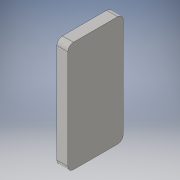
# Autodesk Inventor part: Phone
Saved by Autodesk Inventor 2016 (Build 200138000, 138)
## iProperties
Created: 2017-01-27
Part Number: Phone
Material: Generic
Document SubType Name: Modeling
Designer: RoboticsUser
Density: 1 g/cm^3
Appearance: Default
Author: RoboticsUser
Autodesk Inventor part; units mm, degrees
ref_plane "YZ Plane" through (0, 0, 0) normal (1, 0, 0) x (0, 1, 0)
ref_plane "XZ Plane" through (0, 0, 0) normal (0, 1, 0) x (-1, 0, 0)
ref_plane "XY Plane" through (0, 0, 0) normal (0, 0, 1) x (1, 0, 0)
sketch "Sketch1" plane through (0, 0, 0) normal (1, 0, 0) x (0, 1, 0)
  line L0 (0, 0) -> (127, 0)
  line L1 (127, 0) -> (127, -63.5)
  line L2 (127, -63.5) -> (0, -63.5)
  line L3 (0, -63.5) -> (0, 0)
  dimension "d0" = 127
  dimension "d1" = 63.5
  constraints: 8 end point, 2 parallel, 1 horizontal, 1 perpendicular
  measures "d0" distance of L1.end L2.end
  measures "d1" distance of L0.end L1.end
extrude "Extrusion1" add sketch "Sketch1" along normal blind 12.7
fillet "Fillet1" radius 6.35 1 edges at (6.35, 127, -63.5)
fillet "Fillet2" radius 6.35 1 edges at (6.35, 127, 0)
fillet "Fillet3" radius 6.35 1 edges at (6.35, 0, 0)
fillet "Fillet4" radius 6.35 1 edges at (6.35, 0, -63.5)
body "Solid1"
